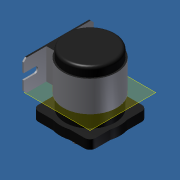
# Autodesk Inventor part: realy
Saved by Autodesk Inventor 2012 (Build 160160000, 160)
## iProperties
Created: 2012-03-25
Part Number: realy
Material: Default
Document SubType Name: Modeling
Designer: Edward
Density: 3.35732 g/cm^3
Mass: 754.097 g
Surface Area: 285.45 cm^2
Volume: 224.613 cm^3
Author: Edward
Autodesk Inventor part; units mm, degrees
ref_plane "YZ Plane" through (0, 0, 0) normal (1, 0, 0) x (0, 1, 0)
ref_plane "XZ Plane" through (0, 0, 0) normal (0, 1, 0) x (-1, 0, 0)
ref_plane "XY Plane" through (0, 0, 0) normal (0, 0, 1) x (1, 0, 0)
sketch "Sketch1" plane through (0, 0, 0) normal (0, 0, 1) x (1, 0, 0)
  line L0 (0, 0) -> (0, 60.96)
  line L1 (0, 60.96) -> (25.4, 60.96)
  arc A0 (28.575, 57.785) -> (25.4, 60.96) centre (25.4, 57.785) ccw
  line L2 (28.575, 57.785) -> (28.575, 0)
  line L3 (28.575, 0) -> (0, 0)
  dimension "d0" = 3.175
  dimension "d1" = 60.96
  dimension "d3" = 28.575
  constraints: 8 end point, 3 perpendicular, 2 point on circle, 2 tangent, 1 centre point, 1 vertical
  measures "d0" radius of A0
  measures "d1" distance between parallel lines of L3 L1
  measures "d3" distance between parallel lines of L2 L0
revolve "Can" add sketch "Sketch1" angle 360 about axis through (0, 0, 0) along (0, 1, 0)
sketch "Sketch2" plane through (0, 0, 0) normal (0, -1, 0) x (1, 0, 0)
  circle A0 centre (0, 0) radius 28.575 projected
  circle A1 centre (0, 0) radius 34.036
  line L0 (-26.3398, 32.6898) -> (26.3398, 32.6898)
  line L1 (32.6898, 26.3398) -> (32.6898, -26.3398)
  line L2 (26.3398, -32.6898) -> (-26.3398, -32.6898)
  line L3 (-32.6898, -26.3398) -> (-32.6898, 26.3398)
  arc A2 (32.6898, 26.3398) -> (26.3398, 32.6898) centre (26.3398, 26.3398) ccw
  arc A3 (-26.3398, 32.6898) -> (-32.6898, 26.3398) centre (-26.3398, 26.3398) ccw
  arc A4 (-32.6898, -26.3398) -> (-26.3398, -32.6898) centre (-26.3398, -26.3398) ccw
  arc A5 (26.3398, -32.6898) -> (32.6898, -26.3398) centre (26.3398, -26.3398) ccw
  point P0 (-32.6898, 32.6898)
  point P1 (32.6898, 32.6898)
  point P2 (0, 32.6898)
  point P3 (-32.6898, 0)
  dimension "d5" = 65.3796
  dimension "d6" = 68.072
  dimension "d7" = 6.35
  constraints: 8 end point, 8 point on circle, 8 tangent, 5 centre point, 4 point on line, 3 equal radius, 2 midpoint, 2 parallel, 2 perpendicular, 1 coincident, 1 horizontal, 1 horizontal alignment, 1 vertical alignment
  measures "d5" distance of point (-32.69, 32.69) point (32.69, 32.69)
  measures "d6" diameter of A1
  measures "d7" radius of A2
extrude "Plate" add sketch "Sketch2" along normal blind 10.3632 contours A0 | A1 L1 | L1 A1 L2 L3 L0 | A1 L0 A2 L1 | L1 A5 L2 A1 | L0 A1 | A1 L2 | A1 L3 A3 L0 | L2 A4 L3 A1 | L3 A1
sketch "Sketch3" plane through (0, -10.3632, 0) normal (0, -1, 0) x (1, 0, 0)
  arc A0 (-9.4777, -32.6898) -> (9.4777, -32.6898) centre (0, 0) ccw projected
  circle A1 centre (-16.1798, 0) radius 2.413
  circle A2 centre (16.1798, 0) radius 2.413
  dimension "d10" = 4.826
  dimension "d11" = 32.3596
  dimension "d12" = 16.1798
  constraints: 2 centre point, 1 equal radius
  measures "d10" diameter of A1
  measures "d11" distance of A2.centre A1.centre
  measures "d12" distance of A1.centre A0.centre
extrude "Coil Studs" add sketch "Sketch3" along normal blind 9.525
thread "Coil Stud 1" size "10-32 UNF" class "2A" standard "ANSI Unified Screw Threads" full length
thread "Coil Stud 2" size "10-32 UNF" class "2A" standard "ANSI Unified Screw Threads" full length
sketch "Sketch4" plane through (0, -10.3632, 0) normal (0, -1, 0) x (1, 0, 0)
  arc A0 (-9.4777, -32.6898) -> (9.4777, -32.6898) centre (0, 0) ccw projected
  circle A1 centre (0, 14.6812) radius 3.9688
  circle A2 centre (0, -14.6812) radius 3.9688
  dimension "d19" = 29.3624
  dimension "d20" = 14.6812
  dimension "d21" = 7.9375
  constraints: 2 centre point, 1 equal radius
  measures "d19" distance of A1.centre A2.centre
  measures "d20" distance of A0.centre A2.centre
  measures "d21" diameter of A1
extrude "Power Studs" add sketch "Sketch4" along normal blind 15.0876
thread "Power Stud 1" size "5/16-18 UNC" class "2A" standard "ANSI Unified Screw Threads" full length
thread "Power Stud 2" size "5/16-18 UNC" class "2A" standard "ANSI Unified Screw Threads" full length
ref_plane "Work Plane1" through (0, 15.24, 0) normal (0, 1, 0) x (1, 0, 0)
sketch "Sketch5" plane through (0, 15.24, 0) normal (0, 1, 0) x (1, 0, 0)
  line L0 (-37.592, 12.4714) -> (-19.05, 12.4714)
  line L1 (-19.05, 12.4714) -> (-19.05, -12.4714)
  line L2 (-19.05, -12.4714) -> (-37.592, -12.4714)
  line L3 (-37.592, -12.4714) -> (-37.592, 12.4714)
  point P0 (0, 0)
  point P1 (-19.05, 0)
  dimension "d29" = 37.592
  dimension "d30" = 24.9428
  dimension "d31" = 19.05
  constraints: 8 end point, 2 parallel, 1 horizontal, 1 horizontal alignment, 1 midpoint, 1 perpendicular
  measures "d29" distance from line of point (0, 0) L3
  measures "d30" distance of L2.end L0.start
  measures "d31" distance from line of point (0, 0) L1
extrude "Extrusion4" add sketch "Sketch5" along normal blind 34.925
sketch "Sketch6" plane through (0, 50.165, 0) normal (0, 1, 0) x (1, 0, 0)
  arc A0 (-25.7098, 12.4714) -> (-25.7098, -12.4714) centre (0, 0) ccw projected
  line L0 (-37.592, 12.4714) -> (-25.7098, 12.4714) projected
  line L1 (-25.7098, -12.4714) -> (-37.592, -12.4714) projected
  line L2 (-37.592, 12.4714) -> (-35.7632, 12.4714)
  line L3 (-35.7632, 13.97) -> (-35.7632, 39.6951)
  line L4 (-35.7632, 39.6951) -> (-37.592, 39.6951)
  line L5 (-37.592, 39.6951) -> (-37.592, 12.4714)
  circle A1 centre (0, 0) radius 28.575
  arc A2 (-26.8755, -13.97) -> (-26.8755, 13.97) centre (0, 0) ccw
  line L6 (-35.7632, 13.97) -> (-26.8755, 13.97)
  line L7 (-37.592, -12.4714) -> (-35.7632, -12.4714)
  line L8 (-35.7632, -13.97) -> (-35.7632, -39.6951)
  line L9 (-35.7632, -39.6951) -> (-37.592, -39.6951)
  line L10 (-37.592, -39.6951) -> (-37.592, -12.4714)
  line L11 (-35.7632, -13.97) -> (-26.8755, -13.97)
  dimension "d34" = 57.15
  dimension "d35" = 60.579
  dimension "d36" = 27.94
  dimension "d37" = 1.8288
  dimension "d38" = 79.3902
  constraints: 20 end point, 4 parallel, 4 perpendicular, 3 equal length, 2 centre point, 2 coincident, 2 horizontal, 2 point on circle
  measures "d34" diameter of A1
  measures "d35" diameter of A2
  measures "d36" distance between parallel lines of L11 L6
  measures "d37" distance of L3.end L4.end
  measures "d38" distance between parallel lines of L9 L4
extrude "Mounting Plate" add sketch "Sketch6" against normal blind 34.925 contours L0 L5 L4 L3 L6 A2 L11 L8 L9 L10 L1 A1
sketch "Sketch7" plane through (-37.592, 15.24, -39.6951) normal (-1, 0, 0) x (0, 0, 1)
  line L0 (0, 34.925) -> (79.3902, 34.925) projected
  line L1 (0, 34.925) -> (0, 0) projected
  line L2 (0, 0) -> (79.3902, 0) projected
  line L3 (79.3902, 34.925) -> (79.3902, 0) projected
  circle A0 centre (12.7, 17.4625) radius 3.5687
  line L4 (0, 21.0312) -> (12.7, 21.0312)
  line L5 (12.7, 21.0312) -> (12.7, 13.8938)
  line L6 (12.7, 13.8938) -> (0, 13.8938)
  line L7 (0, 13.8938) -> (0, 21.0312)
  line L8 (0, 31.75) -> (3.175, 34.925)
  line L9 (0, 17.4625) -> (79.3902, 17.4625)
  line L10 (39.6951, 34.925) -> (39.6951, 0)
  circle A1 centre (66.6902, 17.4625) radius 3.5687
  line L11 (79.3902, 21.0312) -> (66.6902, 21.0312)
  line L12 (66.6902, 21.0312) -> (66.6902, 13.8938)
  line L13 (66.6902, 13.8938) -> (79.3902, 13.8938)
  line L14 (79.3902, 13.8938) -> (79.3902, 21.0312)
  line L15 (0, 3.175) -> (3.175, 0)
  line L16 (79.3902, 3.175) -> (76.2152, 0)
  line L17 (76.2152, 34.925) -> (79.3902, 31.75)
  point P0 (39.6951, -15.24)
  dimension "d41" = 7.1374
  dimension "d42" = 12.7
  dimension "d43" = 3.175
  dimension "d44" = 3.175
  constraints: 28 end point, 9 point on line, 7 perpendicular, 5 midpoint, 5 symmetric about line, 3 horizontal, 2 parallel, 2 vertical alignment, 1 vertical, 4 other
  measures "d41" distance between parallel lines of L4 L6
  measures "d42" distance of L4.start L4.end
  measures "d43" horizontal distance of L8.start L8.end
  measures "d44" horizontal distance of L8.start L8.end
extrude "Extrusion6" cut sketch "Sketch7" against normal up to next contours L0 L8 L1 | L4 A0 L9 L1 | L0 L3 L17 | L9 A0 L6 L1 | L5 L9 A0 | A0 L9 L5 | A0 L5 L9 | A1 L12 L9 | L9 L12 A1 | L9 L5 A0 | L3 L9 A1 L11 | L12 A1 L9 | L9 A1 L12 | A1 L9 L3 L13 | L2 L1 L15 | L16 L3 L2
equation "\"d12\" = 0.5 * d11"
equation "\"d20\" = 0.5 * d19"
body "Solid1"
